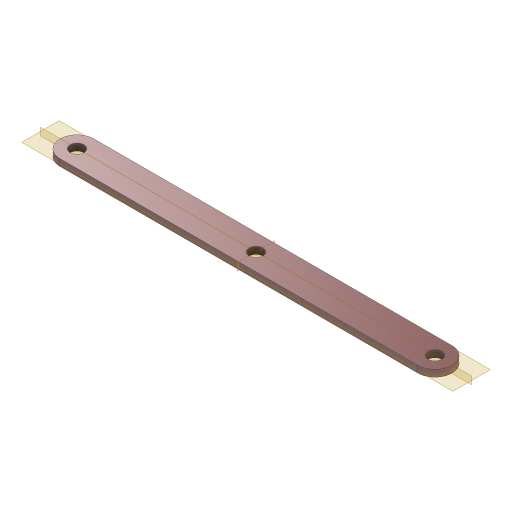
# Autodesk Inventor part: Рельс платформы подъёмника
Saved by Autodesk Inventor 2023.2 (Build 272271030, 271C)
## iProperties
Created: 2025-03-18
Part Number: Рельс платформы подъёмника
Material: Типовые
Document SubType Name: Modeling
Designer: Коноваленко
Density: 1 g/cm^3
Appearance: По умолчанию
Author: Коноваленко
Autodesk Inventor part; units mm, degrees
sketch "Эскиз1" plane through (0, 0, 0) normal (0, 1, 0) x (-1, 0, 0)
  line L0 (105, 10) -> (-105, 10)
  line L1 (-105, -10) -> (105, -10)
  line L2 (105, 10) -> (-105, -10) construction
  line L3 (-105, 10) -> (105, -10) construction
  arc A0 (-105, 10) -> (-105, -10) centre (-105, 0) ccw
  arc A1 (105, -10) -> (105, 10) centre (105, 0) ccw
  line L4 (0, -14) -> (0, 14) construction
  circle A2 centre (105, 0) radius 4
  circle A3 centre (-105, 0) radius 4
  circle A4 centre (0, 0) radius 4
  line L5 (-161, 0) -> (161, 0) projected
  point P0 (0, 10)
  point P1 (0, -10)
  dimension "d2" = 210
  dimension "d5" = 8
  dimension "d6" = 8
  dimension "d9" = 8
  dimension "d17" = 10
  constraints: 8 end point, 5 centre point, 4 point on circle, 3 coincident, 2 midpoint, 2 tangent, 1 horizontal, 1 parallel, 1 point on line
  measures "d2" distance of L1.start L1.end
  measures "d5" diameter of A2
  measures "d6" diameter of A3
  measures "d9" diameter of A4
  measures "d17" distance of L1.end A1.centre
extrude "Выдавливание1" add sketch "Эскиз1" along normal mid plane 4 contours A1 L5 A2 A4 A3 A0 L0 | A1 L1 A0 L5 A3 A4 A2
